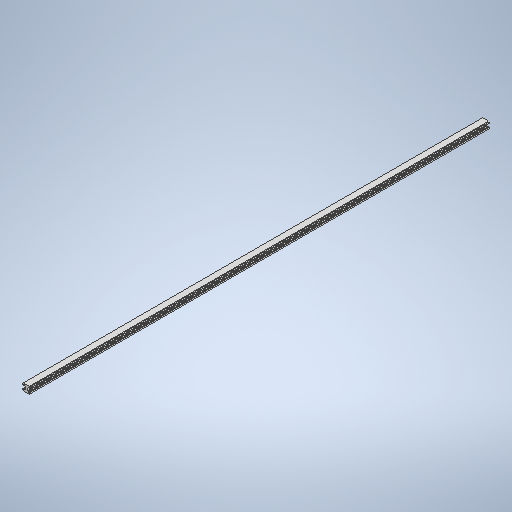
# Autodesk Inventor part: profile_0001_0001
Saved by Autodesk Inventor 2025.2 (Build 292293000, 293)
## iProperties
Created: 2025-03-25
Part Number: profile_0001_0001
Material: Generic
Document SubType Name: Modeling
Designer: kenne
Density: 1 g/cm^3
Appearance: Default
Author: kenne
Autodesk Inventor part; units mm, degrees
ref_plane "YZ Plane" through (0, 0, 0) normal (1, 0, 0) x (0, 1, 0)
ref_plane "XZ Plane" through (0, 0, 0) normal (0, 1, 0) x (-1, 0, 0)
ref_plane "XY Plane" through (0, 0, 0) normal (0, 0, 1) x (1, 0, 0)
sketch "Sketch1" plane through (0, 0, 0) normal (0, 0, 1) x (1, 0, 0)
  line L0 (-7.5, 7.5) -> (7.5, 7.5) construction
  line L1 (-7.5, 7.5) -> (-7.5, 3.1) construction
  line L2 (-7.5, 3.1) -> (-5.5, 3.1) construction
  line L3 (-5.5, 5.6) -> (-5.5, 3.1) construction
  line L4 (-5.5, 5.6) -> (-3, 3.1) construction
  line L5 (-3, 0) -> (0, 0)
  line L6 (0, 0) -> (0, 7.5)
  arc A0 (-6.5, 7.5) -> (-7.5, 6.5) centre (-6.5, 6.5) ccw
  line L7 (-7.5, 6.5) -> (-7.5, 3.1) construction
  line L8 (-6.5, 7.5) -> (0, 7.5)
  arc A1 (-4.6464, 4.7464) -> (-5.5, 4.3929) centre (-5, 4.3929) ccw
  line L9 (-5.5, 4.3929) -> (-5.5, 3.1)
  line L10 (-3, 3.1) -> (-3, 0) construction
  arc A2 (-3, 2.8929) -> (-3.1464, 3.2464) centre (-3.5, 2.8929) ccw
  line L11 (-4.6464, 4.7464) -> (-3.1464, 3.2464)
  line L12 (-3, 2.8929) -> (-3, 0)
  line L13 (-7.5, 3.1) -> (-7, 3.1) construction
  line L14 (-7, 3.1) -> (-7, 3.6)
  line L15 (-7, 3.6) -> (-7.5, 3.6)
  line L16 (-7.5, 3.6) -> (-7.5, 3.1) construction
  line L17 (-7.5, 6.5) -> (-7.5, 3.6)
  line L18 (-5.5, 3.1) -> (-7, 3.1)
  dimension "d0" = 15
  dimension "d1" = 7.5
  dimension "d3" = 2
  dimension "d4" = 2.5
  dimension "d5" = 45
  dimension "d9" = 1
  dimension "d10" = 0.5
  dimension "d11" = 0.5
  dimension "d12" = 0.5
  dimension "d13" = 3.1
  constraints: 38 end point, 6 point on circle, 6 point on line, 6 tangent, 4 horizontal, 3 centre point, 3 perpendicular, 3 vertical, 2 horizontal alignment, 2 parallel, 1 midpoint, 1 vertical alignment
  measures "d0" distance of L0.start L0.end
  measures "d1" distance of L5.end L6.end
  measures "d3" distance of L1.end L2.end
  measures "d4" distance of L3.start L2.end
  measures "d5" angle of L3 L4
  measures "d9" radius of A0
  measures "d10" radius of A1
  measures "d11" radius of A2
  measures "d12" distance of L14.end L15.end
  measures "d13" distance from line of L5.end L2
extrude "Extrusion1" add sketch "Sketch1" against normal blind 1000
mirror "Mirror3" about plane through (0, 0, 0) normal (1, 0, 0) of "Extrusion1"
mirror "Mirror4" about plane through (0, 0, 0) normal (0, 1, 0) of "Extrusion1", "Mirror3"
equation "\"d1\" = 0.5 * d0"
body "Solid1"
